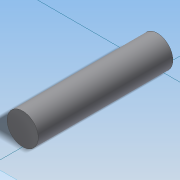
# Autodesk Inventor part: 4mm bullet female
Saved by Autodesk Inventor 2014 SP2 (Build 180246200, 246)
## iProperties
Created: 2014-06-06
Part Number: 4mm bullet female
Material: Generic
Document SubType Name: Modeling
Designer: dliu
Density: 1 g/cm^3
Appearance: Default
Author: dliu
Autodesk Inventor part; units mm, degrees
ref_plane "YZ Plane" through (0, 0, 0) normal (1, 0, 0) x (0, 1, 0)
ref_plane "XZ Plane" through (0, 0, 0) normal (0, 1, 0) x (-1, 0, 0)
ref_plane "XY Plane" through (0, 0, 0) normal (0, 0, 1) x (1, 0, 0)
sketch "Sketch1" plane through (0, 0, 0) normal (0, 0, 1) x (1, 0, 0)
  circle A0 centre (0, 0) radius 2.3813
  dimension "d0" = 4.7625
  constraints: 1 centre point
  measures "d0" diameter of A0
extrude "Extrusion1" add sketch "Sketch1" along normal blind 20.5867
sketch "Sketch2" plane through (0, 0, 0) normal (0, 0, 1) x (1, 0, 0)
  circle A0 centre (0, 0) radius 1.9939
  dimension "d3" = 3.9878
  constraints: 1 centre point
  measures "d3" diameter of A0
extrude "Extrusion2" cut sketch "Sketch2" along normal blind 14.1986
body "Solid1"
